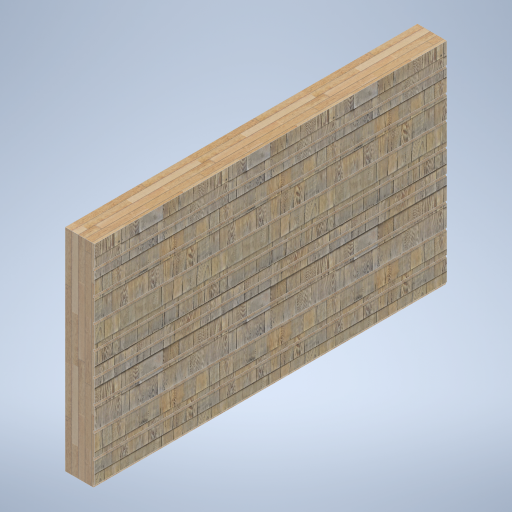
# Autodesk Inventor part: side_wall_block_02
Saved by Autodesk Inventor 2024.2 (Build 282272000, 272)
## iProperties
Created: 2024-05-22
Part Number: side_wall_block_02
Material: Wood (Maple)
Document SubType Name: Modeling
Designer: LOSTER_1
Density: 0.67 g/cm^3
Appearance: Natural Maple - Glossy Dark Tint
Author: LOSTER_1
Autodesk Inventor part; units mm, degrees
ref_plane "YZ Plane" through (0, 0, 0) normal (1, 0, 0) x (0, 1, 0)
ref_plane "XZ Plane" through (0, 0, 0) normal (0, 1, 0) x (-1, 0, 0)
ref_plane "XY Plane" through (0, 0, 0) normal (0, 0, 1) x (1, 0, 0)
sketch "Sketch1" plane through (0, 0, 0) normal (1, 0, 0) x (0, 1, 0)
  line L0 (-1801.9397, -1488.283) -> (-1801.9397, 1511.717)
  line L1 (-1.6085, 1511.717) -> (-1801.9397, 1511.717)
  line L2 (-1801.9397, -1488.283) -> (-1.6085, -1488.283)
  line L3 (-1.6085, 1511.717) -> (-1.6085, -1488.283)
  point P0 (0, 0)
  constraints: 8 end point, 1 vertical
extrude "Extrusion1" add sketch "Sketch1" along normal blind 250
sketch "Sketch2" plane through (0, -1801.9397, 1511.717) normal (0, 0, 1) x (1, 0, 0)
  line L0 (0, 0) -> (250, 0) projected
  line L1 (250, 1800.3312) -> (250, 0) projected
  line L2 (0, 1800.3312) -> (250, 1800.3312) projected
  line L3 (0, 1800.3312) -> (250, 1800.3312) projected
  line L4 (0, 1800.3312) -> (250, 1800.3312)
  line L5 (250, 1800.3312) -> (250, 1620.3312)
  line L6 (250, 0) -> (250, 1800.3312) projected
  line L7 (250, 1620.3312) -> (240.3332, 1620.3312)
  line L8 (240.3332, 1620.3312) -> (240.3332, 1600.3312)
  line L9 (240.3332, 1600.3312) -> (250, 1600.3312)
  line L10 (250, 1600.3312) -> (250, 1420.3312)
  line L11 (250, 1420.3312) -> (240.3332, 1420.3312)
  line L12 (240.3332, 1420.3312) -> (240.3332, 1400.4363)
  line L13 (240.3332, 1400.4363) -> (250, 1400.4363)
  line L14 (250, 1400.4363) -> (250, 1220.4363)
  line L15 (250, 1220.4363) -> (240.3332, 1220.4363)
  line L16 (240.3332, 1220.4363) -> (240.3332, 1200.6098)
  line L17 (240.3332, 1200.6098) -> (250, 1200.6098)
  line L18 (250, 1200.6098) -> (250, 1020.6098)
  line L19 (250, 1020.6098) -> (240.3332, 1020.6098)
  line L20 (240.3332, 1020.6098) -> (240.3332, 1000.7833)
  line L21 (240.3332, 1000.7833) -> (250, 1000.7833)
  line L22 (250, 1000.7833) -> (250, 820.7833)
  line L23 (250, 820.7833) -> (240.3332, 820.7833)
  line L24 (240.3332, 820.7833) -> (240.3332, 800.7425)
  line L25 (240.3332, 800.7425) -> (250, 800.7425)
  line L26 (250, 800.7425) -> (250, 620.7425)
  line L27 (250, 620.7425) -> (240.3332, 620.7425)
  line L28 (240.3332, 620.7425) -> (240.3332, 600.7016)
  line L29 (240.3332, 600.7016) -> (250, 600.7016)
  line L30 (250, 600.7016) -> (250, 420.7016)
  line L31 (250, 420.7016) -> (240.3332, 420.7016)
  line L32 (240.3332, 420.7016) -> (240.3332, 400.4572)
  line L33 (240.3332, 400.4572) -> (250, 400.4572)
  line L34 (250, 400.4572) -> (250, 220.4572)
  line L35 (250, 220.4572) -> (240.3332, 220.4572)
  line L36 (240.3332, 220.4572) -> (240.3332, 200.4261)
  line L37 (240.3332, 200.4261) -> (250, 200.4261)
  line L38 (250, 200.4261) -> (250, 20.0398)
  line L39 (240.3332, 20.0398) -> (240.3332, 0)
  line L40 (240.3332, 20.0398) -> (250, 20.0398)
  line L41 (250, 0) -> (240.3332, 0)
  line L42 (250, 0.5032) -> (250, 1620.3312)
  point P0 (0, 1801.9397)
  dimension "d2" = 180
  dimension "d3" = 20
  dimension "d4" = 180
  dimension "d5" = 180
  dimension "d6" = 180
  dimension "d7" = 180
  dimension "d8" = 180
  dimension "d9" = 180
  dimension "d10" = 180
  constraints: 76 end point, 19 point on line, 13 horizontal, 6 perpendicular, 1 parallel, 1 vertical, 17 other
  measures "d2" distance of L2.end L5.end
  measures "d3" distance of L7.end L8.end
  measures "d4" distance of L9.end L10.end
  measures "d5" distance of L13.end L14.end
  measures "d6" distance of L17.end L18.end
  measures "d7" distance of L21.end L22.end
  measures "d8" distance of L25.end L26.end
  measures "d9" distance of L29.end L30.end
  measures "d10" distance of L33.end L34.end
extrude "Extrusion2" cut sketch "Sketch2" against normal through all
body "Solid1"
